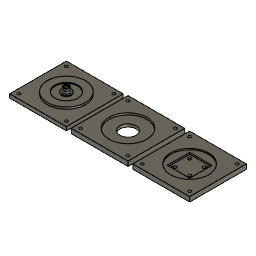
AS5600 holder v1.1 (Autodesk Fusion 360 design; units mm, degrees)
part number: 2026-01-20-22-25-40-409
Autodesk Fusion 360 part; units mm, degrees
sketch "Sketch1" plane through (0, 0, 0) normal (0, 0, 1) x (1, 0, 0)
  circle A0 centre (0, 0) radius 1.9
  circle A1 centre (0, 0) radius 4.9
  circle A2 centre (0, 0) radius 20
  dimension "d1" = 3.8
  dimension "d2" = 9.8
  constraint coincident A0.centre A1.centre
  constraint concentric A0 A1
  constraint concentric A1 A2
  measures "d1" diameter of A0
  measures "d2" diameter of A1
sketch "Sketch2" plane through (0, 0, 0) normal (0, 0, 1) x (1, 0, 0)
  line L0 (30, -30) -> (-30, -30)
  line L1 (-30, -30) -> (-30, 30)
  line L2 (-30, 30) -> (30, 30)
  line L3 (30, 30) -> (30, -30)
  line L4 (30, -30) -> (-30, 30) construction
  line L5 (-30, -30) -> (30, 30) construction
  constraint horizontal L0
  constraint perpendicular L0 L1
  constraint parallel L0 L2
  constraint parallel L1 L3
  constraint coincident L4 origin
  constraint coincident L5 origin
extrude "Extrude1" add sketch "Sketch1" along normal blind 5 contours A0 | A1 | A2 makes body 1
sketch "Sketch3" plane through (0, 0, 0) normal (0, 0, 1) x (1, 0, 0)
extrude "Extrude2" add sketch "Sketch2" along normal blind 3 bodies 1
extrude "Extrude3" add sketch "Sketch1" along normal blind 8 contours A0 | A1 bodies 1
sketch "Sketch4" plane through (0, 0, 0) normal (0, 0, 1) x (1, 0, 0)
  circle A0 centre (0, 0) radius 1.9
  dimension "d9" = 3.8
  constraint coincident A0.centre origin
  measures "d9" diameter of A0
sketch "Sketch5" plane through (0, 0, 8) normal (0, 0, 1) x (-1, 0, 0)
  circle A0 centre (0, 0) radius 4.9
  circle A1 centre (0, 0) radius 1.9
  dimension "d10" = 3.8
  constraint coincident A0.centre A1.centre
  measures "d10" diameter of A1
extrude "Extrude4" cut sketch "Sketch5" against normal blind 1 contours A1 bodies 1
sketch "Sketch6" plane through (0, 0, 3) normal (0, 0, 1) x (-1, 0, 0)
  line L0 (-30, -30) -> (30, -30)
  line L1 (30, -30) -> (30, 30)
  line L2 (30, 30) -> (-30, 30)
  line L3 (-30, 30) -> (-30, -30)
  circle A0 centre (0, 0) radius 20
  line L4 (-11.75, -11.75) -> (11.75, -11.75)
  line L5 (11.75, -11.75) -> (11.75, 11.75)
  line L6 (11.75, 11.75) -> (-11.75, 11.75)
  line L7 (-11.75, 11.75) -> (-11.75, -11.75)
  line L8 (-11.75, -11.75) -> (11.75, 11.75) construction
  line L9 (11.75, -11.75) -> (-11.75, 11.75) construction
  line L10 (11.75, -11.75) -> (8.75, -11.75)
  line L11 (8.75, -11.75) -> (8.75, -8.75)
  line L12 (8.75, -8.75) -> (11.75, -8.75)
  line L13 (11.75, -8.75) -> (11.75, -11.75)
  line L14 (-8.75, -11.75) -> (-11.75, -11.75)
  line L15 (-11.75, -11.75) -> (-11.75, -8.75)
  line L16 (-8.75, -8.75) -> (-8.75, -11.75)
  line L17 (-11.75, -8.75) -> (-8.75, -8.75)
  line L18 (11.75, 8.75) -> (8.75, 8.75)
  line L19 (8.75, 8.75) -> (8.75, 11.75)
  line L20 (11.75, 11.75) -> (11.75, 8.75)
  line L21 (8.75, 11.75) -> (11.75, 11.75)
  line L22 (-8.75, 8.75) -> (-11.75, 8.75)
  line L23 (-11.75, 8.75) -> (-11.75, 11.75)
  line L24 (-8.75, 11.75) -> (-8.75, 8.75)
  line L25 (-11.75, 11.75) -> (-8.75, 11.75)
  circle A1 centre (8.75, -8.75) radius 1.0607
  circle A2 centre (-8.75, -8.75) radius 1.0607
  circle A3 centre (8.75, 8.75) radius 1.0607
  circle A4 centre (-8.75, 8.75) radius 1.0607
  dimension "d13" = 23.5
  dimension "d14" = 23.5
  dimension "d15" = 3
  dimension "d16" = 3
  constraint horizontal L4
  constraint perpendicular L4 L5
  constraint parallel L4 L6
  constraint parallel L5 L7
  constraint coincident L8 A0.centre
  constraint coincident L9 A0.centre
  constraint coincident A0.centre origin
  constraint horizontal L10
  constraint vertical L11
  constraint horizontal L12
  constraint vertical L13
  constraint coincident L11.end L12.start
  measures "d13" distance of L4.start L4.end
  measures "d14" distance of L4.start L6.end
  measures "d15" distance of L10.end L11.end
  measures "d16" distance of L11.end L12.end
copy_body "CopyPasteBodies1" bodies 1 makes body 2
move_body "Move1" bodies 2 to x (1, 0, 0) y (0, 1, 0) z (0, 0, 1) at (80, 0, 0)
extrude "Extrude5" add 1 faces at (14.874, -1.2371, 5) along direction (0, 0, 1) blind 3 on bodies 1 bodies 1
extrude "Extrude6" cut 1 faces at (13.8922, -0.9936, 8) along direction (0, 0, -1) blind 4.8 on bodies 1 bodies 1
extrude "Extrude7" cut 1 faces at (-0.5831, 0.5093, 7) along direction (0, 0, -1) blind 3.85 on bodies 1 bodies 1
extrude "Extrude8" cut sketch "Sketch6" against normal blind 4 contours L16 L17 A2 | L16 L17 A2 | L11 L12 A1 | L11 L12 A1 | L22 L24 A4 | L22 L24 A4 | L18 L19 A3 | L18 L19 A3 bodies 1
extrude "Extrude9" cut 4 faces at (-8.8616, -8.364, 3) (8.5801, -9.0108, 3) (8.4908, 9.1677, 3) (-9.256, 9.0666, 3) along direction (0, 0, 1) blind 4 on bodies 1 bodies 1
extrude "Extrude10" cut 1 faces at (-12.7583, 0, 3.2) along direction (0, 0, -1) blind 0.5 on bodies 1 bodies 1
extrude "Extrude11" cut 1 faces at (-0.5831, 0.5093, 3.15) along direction (0, 0, -1) blind 1 on bodies 1 bodies 1
extrude "Extrude12" cut sketch "Sketch6" against normal blind 1 contours L4 L7 L14 L15 L16 L17 A2 | L4 L5 L6 L7 L11 L12 L16 L17 L18 L19 L22 L24 A1 A2 A3 A4 | L4 L5 L10 L11 L12 L13 A1 | L6 L7 L22 L23 L24 L25 A4 | L5 L6 L18 L19 L20 L21 A3 bodies 1
extrude "Extrude13" cut 1 faces at (83.8818, -0.2434, 8) along direction (0, 0, -1) blind 3 on bodies 2 bodies 2
sketch "Sketch7" plane through (0, 0, 7) normal (0, 0, 1) x (-1, 0, 0)
  circle A0 centre (-80, 0) radius 1.9
  circle A1 centre (-80, 0) radius 3.05
  dimension "d44" = 6.1
  constraint concentric A0 A1
  measures "d44" diameter of A1
extrude "Extrude14" add sketch "Sketch7" against normal blind 2 bodies 2
sketch "Sketch8" plane through (0, 0, 7) normal (0, 0, 1) x (-1, 0, 0)
  circle A0 centre (-80, 0) radius 3.05
  circle A1 centre (-80, 0) radius 1.95
  constraint concentric A0 A1
extrude "Extrude15" add sketch "Sketch8" along normal blind 5 bodies 2
extrude "Extrude16" cut 1 faces at (80.8351, 2.5426, 12) along direction (0, 0, -1) blind 1 on bodies 2 bodies 2
extrude "Extrude17" cut 1 faces at (80.8351, 2.5426, 11) along direction (0, 0, -1) blind 0.5 on bodies 2 bodies 2
extrude "Extrude18" add 1 faces at (79.4144, 0.282, 7) along direction (0, 0, 1) blind 2.5 on bodies 2 bodies 2
sketch "Sketch9" plane through (0, 0, 3) normal (0, 0, 1) x (-1, 0, 0)
  line L0 (-30, -30) -> (30, -30)
  line L1 (30, -30) -> (30, 30)
  line L2 (30, 30) -> (-30, 30)
  line L3 (-30, 30) -> (-30, -30)
  circle A0 centre (0, 0) radius 20
  circle A1 centre (0, 0) radius 8.25
  dimension "d55" = 16.5
  constraint concentric A0 A1
  measures "d55" diameter of A1
copy_body "CopyPasteBodies2" bodies 2 makes body 3
move_body "Move2" bodies 3 to x (1, 0, 0) y (0, 1, 0) z (0, 0, 1) at (85, 0, 0)
extrude "Extrude19" cut 1 faces at (162.328, 0.1515, 10.5) along direction (0, 0, -1) blind 2 on bodies 3 bodies 3
move_face "OffsetFaces1" offset -5 1 faces at (164.4144, 0.282, 9.5) on bodies 3
move_face "OffsetFaces2" offset -3.5 1 faces at (162.328, 0.1515, 8.5) on bodies 3
extrude "Extrude20" cut 1 faces at (178.9016, -1.0905, 5) along direction (0, 0, -1) blind 2 on bodies 3 bodies 3
extrude "Extrude21" cut 1 faces at (164.4144, 0.282, 4.5) along direction (0, 0, -1) blind 1.5 on bodies 3 bodies 3
sketch "Sketch10" plane through (0, 0, 3) normal (0, 0, 1) x (-1, 0, 0)
  line L0 (-195, -30) -> (-135, -30)
  line L1 (-135, -30) -> (-135, 30)
  line L2 (-135, 30) -> (-195, 30)
  line L3 (-195, 30) -> (-195, -30)
  circle A0 centre (-165, 0) radius 8.525
  circle A1 centre (-165, 0) radius 20
  dimension "d67" = 17.05
  constraint concentric A0 A1
  measures "d67" diameter of A0
extrude "Extrude22" cut sketch "Sketch10" against normal blind 7 contours A0 bodies 3
extrude "Extrude23" add sketch "Sketch10" along normal blind 2 contours A1 bodies 3
extrude "Extrude24" add 1 faces at (148.9312, 1.4171, 5) along direction (0, 0, 1) blind 1 on bodies 3 bodies 3
sketch "Sketch11" plane through (0, 0, 3) normal (0, 0, 1) x (1, 0, 0)
extrude "Extrude25" cut 1 faces at (148.9312, 1.4171, 6) along direction (0, 0, -1) blind 5 on bodies 3 bodies 3
extrude "Extrude26" add sketch "Sketch10" along normal blind 2 contours L0 L1 L2 L3 bodies 3
extrude "Extrude27" add sketch "Sketch10" along normal blind 1 contours A1 bodies 3
move_face "OffsetFaces3" offset -1 1 faces at (148.9312, 1.4171, 4) on bodies 3
extrude "Extrude28" add 1 faces at (148.9312, 1.4171, 1) along direction (0, 0, 1) blind 1 on bodies 3 bodies 3
move_body "Move3" bodies 3 to x (1, 0, 0) y (0, 1, 0) z (0, 0, 1) at (-165, 0, 3)
sketch "Sketch12" plane through (0, 0, 8) normal (0, 0, 1) x (-1, 0, 0)
  circle A0 centre (0, 0) radius 20
  line L0 (-30, 30) -> (-30, -30)
  line L1 (-30, -30) -> (30, -30)
  line L2 (30, -30) -> (30, 30)
  line L3 (30, 30) -> (-30, 30)
  circle A1 centre (-25, 25) radius 1.5
  circle A2 centre (25, 25) radius 1.5
  circle A3 centre (-25, -25) radius 1.5
  circle A4 centre (25, -25) radius 1.5
  dimension "d88" = 50
  dimension "d89" = -50
extrude "Extrude29" cut sketch "Sketch12" against normal blind 14 contours A1 | A2 | A3 | A4 bodies 1 3
sketch "Sketch13" plane through (0, 0, 3) normal (0, 0, 1) x (-1, 0, 0)
  line L0 (-110, -30) -> (-50, -30)
  line L1 (-50, -30) -> (-50, 30)
  line L2 (-50, 30) -> (-110, 30)
  line L3 (-110, 30) -> (-110, -30)
  circle A0 centre (-80, 0) radius 20
  circle A1 centre (-105, 25) radius 1.5
  circle A2 centre (-55, 25) radius 1.5
  circle A3 centre (-105, -25) radius 1.5
  circle A4 centre (-55, -25) radius 1.5
  dimension "d94" = 50
  dimension "d95" = -50
extrude "Extrude30" cut sketch "Sketch13" against normal blind 21 contours A1 | A2 | A3 | A4 bodies 2
move_body "Move4" bodies 2 to x (0, -1, 0) y (1, 0, 0) z (0, 0, 1) at (80, 80, 0)
move_body "Move5" bodies 2 to x (1, 0, 0) y (0, 1, 0) z (0, 0, 1) at (-80, 0, 13)
move_body "Move6" bodies 2 to x (1, 0, 0) y (0, -1, 0) z (0, 0, -1) at (0, -60, 16)
move_body "Move7" bodies 2 to x (1, 0, 0) y (0, 1, 0) z (0, 0, 1) at (0, 60, 8)
move_body "Move8" bodies 2 to x (1, 0, 0) y (0, 1, 0) z (0, 0, 1) at (0, 0, 3)
move_body "Move9" bodies 2 to x (1, 0, 0) y (0, 1, 0) z (0, 0, 1) at (0, 0, 1)
extrude "Extrude31" add 1 faces at (0.4982, -24.1807, 3) along direction (0, 0, 1) blind 1 on bodies 1 bodies 1
extrude "Extrude32" add 1 faces at (-16.0688, 1.4171, 5) along direction (0, 0, 1) blind 1 on bodies 3 bodies 3
move_body "Move10" bodies 1 to x (1, 0, 0) y (0, 1, 0) z (0, 0, 1) at (0, 0, -1)
move_face "MoveFace1" by (0, 0, -1) 1 faces at (-0.9936, 14.2755, 10) on bodies 2
move_body "Move11" bodies 2 to x (1, 0, 0) y (0, 1, 0) z (0, 0, 1) at (0, 0, 3)
move_face "OffsetFaces4" offset 1 1 faces at (-24.1807, 0.4982, 15) on bodies 2
move_body "Move12" bodies 2 to x (1, 0, 0) y (0, 1, 0) z (0, 0, 1) at (0, 0, -5)
move_body "Move13" bodies 1 to x (1, 0, 0) y (0, 1, 0) z (0, 0, 1) at (0, 0, -1)
move_face "OffsetFaces5" offset 1 1 faces at (20.2849, -2.8074, -2) on bodies 1
extrude "Extrude33" cut 1 faces at (2.6575, 2.6762, 0) along direction (0, 0, -1) blind 1 on bodies 1 bodies 1
move_body "Move14" bodies 1 to x (1, 0, 0) y (0, 1, 0) z (0, 0, 1) at (65, 0, 0)
move_body "Move15" bodies 2 to x (1, 0, 0) y (0, 1, 0) z (0, 0, 1) at (-70, 0, 0)
move_body "Move16" bodies 2 to x (-1, 0, 0) y (0, 1, 0) z (0, 0, -1) at (-200, 0, 26)
move_body "Move17" bodies 3 to x (1, 0, 0) y (0, 1, 0) z (0, 0, 1) at (0, 0, -6)
move_body "Move18" bodies 2 to x (1, 0, 0) y (0, 1, 0) z (0, 0, 1) at (60, 0, -16)
move_body "Move19" bodies 2 to x (1, 0, 0) y (0, 1, 0) z (0, 0, 1) at (5, 0, 0)
sketch "Sketch14" plane through (0, 0, 6.5) normal (0, 0, 1) x (-1, 0, 0)
  circle A0 centre (65, 0) radius 1.95
  circle A1 centre (65, 0) radius 2.1
  dimension "d151" = 4.2
  constraint concentric A0 A1
  measures "d151" diameter of A1
extrude "Extrude34" cut sketch "Sketch14" along normal blind 2.8 bodies 2
fillet "Fillet1" radius 0.2 1 edges at (-63.0421, -0.7594, 7.5) on bodies 2
move_face "OffsetFaces6" offset -0.5 1 faces at (-65.5746, -0.8842, 6.5) on bodies 2
sketch "Sketch15" plane through (0, 0, 7.5) normal (0, 0, 1) x (-1, 0, 0)
  circle A0 centre (65, 0) radius 3.05
  circle A1 centre (65, 0) radius 2.3
  circle A2 centre (65, 0) radius 3.15
  constraint concentric A0 A2
move_body "Move20" bodies 2 to x (1, 0, 0) y (0, 1, 0) z (0, 0, 1) at (0, 0, 5)
extrude "Extrude35" add sketch "Sketch15" along normal blind 3 contours A0 | A1 | A2 bodies 2
sketch "Sketch16" plane through (0, 0, 8) normal (0, 0, 1) x (-1, 0, 0)
  circle A0 centre (65, 0) radius 3.15
  circle A1 centre (65, 0) radius 20
  circle A2 centre (65, 0) radius 5.05
  circle A3 centre (65, 0) radius 12
  dimension "d162" = 10.1
  constraint concentric A0 A2
  constraint concentric A2 A3
  measures "d162" diameter of A2
extrude "Extrude36" cut sketch "Sketch16" against normal blind 1 contours A3 bodies 2
move_body "Move21" bodies 2 to x (1, 0, 0) y (0, 1, 0) z (0, 0, 1) at (0, 0, -5)
sketch "Sketch17" plane through (0, 0, -1) normal (0, 0, 1) x (-1, 0, 0)
  circle A0 centre (-56.25, 8.75) radius 1.0607
  circle A1 centre (-56.25, -8.75) radius 1.0607
  circle A2 centre (-73.75, 8.75) radius 1.0607
  circle A3 centre (-73.75, -8.75) radius 1.0607
  line L0 (-76.75, 11.75) -> (-76.75, -11.75)
  line L1 (-76.75, -11.75) -> (-53.25, -11.75)
  line L2 (-53.25, -11.75) -> (-53.25, 11.75)
  line L3 (-53.25, 11.75) -> (-76.75, 11.75)
  circle A4 centre (-57.5, 7.5) radius 1.5
  circle A5 centre (-72.5, 7.5) radius 1.5
  circle A6 centre (-57.5, -7.5) radius 1.5
  circle A7 centre (-72.5, -7.5) radius 1.5
  dimension "d170" = -15
  dimension "d171" = -15
extrude "Extrude37" cut sketch "Sketch17" against normal blind 8 contours A0 A4 | A1 A6 | A2 A5 | A3 A7 picked at (-58.0875, 7.0141) picked at (-58.0875, -7.0141) picked at (-71.9781, 6.9463) picked at (-71.9781, -6.9463) bodies 1
